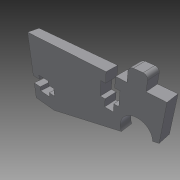
# Autodesk Inventor part: x_carryage_brace_bottom
Saved by Autodesk Inventor 2014 (Build 180170000, 170)
## iProperties
Created: 2014-03-27
Part Number: x_carryage_brace_bottom
Material: Generic
Document SubType Name: Modeling
Designer: buben
Density: 1 g/cm^3
Appearance: Default
Author: buben
Autodesk Inventor part; units mm, degrees
ref_plane "YZ Plane" through (0, 0, 0) normal (1, 0, 0) x (0, 1, 0)
ref_plane "XZ Plane" through (0, 0, 0) normal (0, 1, 0) x (-1, 0, 0)
ref_plane "XY Plane" through (0, 0, 0) normal (0, 0, 1) x (1, 0, 0)
sketch "Sketch1" plane through (0, 0, 0) normal (0, 1, 0) x (-1, 0, 0)
  line L0 (0, -37.5) -> (0, 0)
  line L1 (0, 0) -> (-74.5, 0)
  line L2 (-74.5, 0) -> (-74.5, -18)
  line L3 (-74.5, -18) -> (-15, -37.5)
  line L4 (-15, -37.5) -> (0, -37.5)
  dimension "d0" = 37.5
  dimension "d1" = 74.5
  dimension "d2" = 18
  dimension "d3" = 15
  constraints: 10 end point, 2 parallel, 1 perpendicular, 1 vertical
  measures "d0" distance of L0.start L0.end
  measures "d1" distance of L0.end L1.end
  measures "d2" distance of L1.end L2.end
  measures "d3" distance of L3.end L0.start
extrude "Extrusion1" add sketch "Sketch1" along normal blind 6.5
sketch "Sketch2" plane through (0, 0, 0) normal (0, -1, 0) x (1, 0, 0)
  line L0 (0, 0) -> (0, -37.5) projected
  line L1 (0, -37.5) -> (15, -37.5) projected
  line L2 (16.3, -23.5) -> (16.3, -28)
  line L3 (0, -28) -> (0, -23.5)
  line L4 (5, -21) -> (12.3, -21)
  line L5 (12.3, -30.5) -> (5, -30.5)
  line L6 (0, -23.5) -> (5, -23.5)
  line L7 (12.3, -23.5) -> (16.3, -23.5)
  line L8 (16.3, -28) -> (12.3, -28)
  line L9 (5, -28) -> (0, -28)
  line L10 (5, -30.5) -> (5, -28)
  line L11 (5, -23.5) -> (5, -21)
  line L12 (12.3, -21) -> (12.3, -23.5)
  line L13 (12.3, -28) -> (12.3, -30.5)
  point P0 (16.3, -25.75)
  dimension "d6" = 4.5
  dimension "d7" = 2.5
  dimension "d8" = 5
  dimension "d9" = 7.3
  dimension "d10" = 4
  dimension "d12" = 14
  constraints: 24 end point, 10 parallel, 6 collinear, 4 perpendicular, 3 horizontal, 1 midpoint
  measures "d6" distance of L2.start L2.end
  measures "d7" distance of L8.end L5.start
  measures "d8" distance of L9.start L3.start
  measures "d9" distance of L5.start L5.end
  measures "d10" distance of L2.end L8.end
  measures "d12" distance between parallel lines of L6 L1
extrude "Extrusion2" cut sketch "Sketch2" against normal through all
sketch "Sketch3" plane through (0, 0, 0) normal (0, -1, 0) x (1, 0, 0)
  line L0 (74.5, -18) -> (74.5, 0) projected
  line L1 (74.5, 0) -> (0, 0) projected
  line L2 (66.5, 0) -> (58.5, 0)
  line L3 (58.5, 0) -> (58.5, 4.5)
  line L4 (60.5, 6.5) -> (64.5, 6.5)
  line L5 (66.5, 4.5) -> (66.5, 0)
  arc A0 (60.5, 6.5) -> (58.5, 4.5) centre (60.5, 4.5) ccw
  arc A1 (66.5, 4.5) -> (64.5, 6.5) centre (64.5, 4.5) ccw
  dimension "d15" = 2
  dimension "d16" = 8
  dimension "d17" = 6.5
  dimension "d18" = 8
  constraints: 8 end point, 4 point on circle, 4 tangent, 2 centre point, 2 parallel, 1 equal radius, 1 horizontal, 1 perpendicular, 1 point on line
  measures "d15" radius of A0
  measures "d16" distance between parallel lines of L5 L3
  measures "d17" distance between parallel lines of L1 L4
  measures "d18" distance between parallel lines of L0 L5
extrude "Extrusion3" add sketch "Sketch3" against normal blind 6.5
sketch "Sketch4" plane through (0, 0, 0) normal (0, -1, 0) x (1, 0, 0)
  line L0 (58.5, 4.5) -> (58.5, 0) projected
  line L1 (58.5, 0) -> (0, 0) projected
  line L2 (48.75, 0) -> (53.25, 0)
  line L3 (53.25, -16.3) -> (48.75, -16.3)
  line L4 (55.75, -5) -> (55.75, -12.3)
  line L5 (46.25, -12.3) -> (46.25, -5)
  line L6 (46.25, -5) -> (48.75, -5)
  line L7 (53.25, -5) -> (55.75, -5)
  line L8 (55.75, -12.3) -> (53.25, -12.3)
  line L9 (48.75, -12.3) -> (46.25, -12.3)
  line L10 (48.75, -16.3) -> (48.75, -12.3)
  line L11 (48.75, -5) -> (48.75, 0)
  line L12 (53.25, 0) -> (53.25, -5)
  line L13 (53.25, -12.3) -> (53.25, -16.3)
  point P0 (51, -16.3)
  dimension "d21" = 4.5
  dimension "d22" = 2.5
  dimension "d23" = 5
  dimension "d24" = 4
  dimension "d25" = 7.3
  dimension "d26" = 7.5
  constraints: 24 end point, 10 parallel, 6 collinear, 4 perpendicular, 3 horizontal, 1 midpoint
  measures "d21" distance of L3.start L3.end
  measures "d22" distance of L9.start L5.start
  measures "d23" distance of L6.end L2.start
  measures "d24" distance of L3.end L9.start
  measures "d25" distance of L5.start L5.end
  measures "d26" distance from line of L0 point (51, -16.3)
extrude "Extrusion4" cut sketch "Sketch4" against normal through all
sketch "Sketch5" plane through (0, 0, 0) normal (0, -1, 0) x (1, 0, 0)
  line L0 (15, -37.5) -> (74.5, -18) projected
  line L1 (74.5, -18) -> (74.5, 0) projected
  line L2 (74.5, 0) -> (66.5, 0) projected
  arc A0 (71.9111, -18.8485) -> (57.845, -23.4584) centre (64.5, -20) ccw
  dimension "d29" = 15
  dimension "d30" = 20
  dimension "d31" = 10
  constraints: 2 point on circle, 2 point on line, 1 centre point
  measures "d29" diameter of A0
  measures "d30" distance from line of L2 A0.centre
  measures "d31" distance from line of L1 A0.centre
extrude "Extrusion5" cut sketch "Sketch5" against normal through all
body "Solid1"
